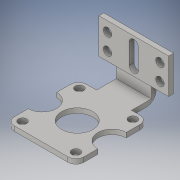
# Autodesk Inventor part: motor mount complete
Saved by Autodesk Inventor 2016 (Build 200138000, 138)
## iProperties
Created: 2017-09-13
Part Number: motor mount complete
Material: Generic
Document SubType Name: Modeling
Designer: student
Density: 1 g/cm^3
Appearance: Default
Author: student
Autodesk Inventor part; units mm, degrees
ref_plane "YZ Plane" through (0, 0, 0) normal (1, 0, 0) x (0, 1, 0)
ref_plane "XZ Plane" through (0, 0, 0) normal (0, 1, 0) x (-1, 0, 0)
ref_plane "XY Plane" through (0, 0, 0) normal (0, 0, 1) x (1, 0, 0)
sketch "Sketch1" plane through (0, 0, 0) normal (0, 0, 1) x (1, 0, 0)
  line L0 (-11.0744, 5.588) -> (11.0744, 5.588)
  line L1 (11.0744, 5.588) -> (11.0744, -5.588)
  line L2 (11.0744, -5.588) -> (-11.0744, -5.588)
  line L3 (-11.0744, -5.588) -> (-11.0744, 5.588)
  circle A0 centre (-8.3312, 2.4384) radius 1.3462
  circle A1 centre (8.3312, 2.4384) radius 1.3462
  circle A2 centre (8.3312, -2.794) radius 1.3462
  circle A3 centre (-8.3312, -2.794) radius 1.3462
  line L4 (0, -3.2143) -> (0, 3.2143) construction
  line L5 (1.4766, -3.2143) -> (1.4766, 3.2143)
  line L6 (-1.4766, 3.2143) -> (-1.4766, -3.2143)
  arc A4 (-1.4766, -3.2143) -> (1.4766, -3.2143) centre (0, -3.2143) ccw
  arc A5 (1.4766, 3.2143) -> (-1.4766, 3.2143) centre (0, 3.2143) ccw
  point P0 (0, 0)
  dimension "d0" = 22.1488
  dimension "d1" = 11.176
  dimension "d2" = 2.6924
  dimension "d3" = 2.6924
  dimension "d4" = 2.6924
  dimension "d5" = 2.6924
  dimension "d6" = 3.1496
  dimension "d7" = 2.794
  dimension "d8" = 5.2324
  dimension "d9" = 2.7432
  dimension "d10" = 2.7432
  dimension "d11" = 3.1496
  dimension "d12" = 2.794
  constraints: 16 end point, 6 centre point, 4 point on circle, 4 tangent, 3 parallel, 2 vertical alignment, 1 horizontal, 1 midpoint, 1 perpendicular, 1 vertical
  measures "d0" distance of L1.end L2.end
  measures "d1" distance of L1.end L0.end
  measures "d2" diameter of A0
  measures "d3" diameter of A1
  measures "d4" diameter of A2
  measures "d5" diameter of A3
  measures "d6" distance from line of L0 A1.centre
  measures "d7" distance from line of L2 A2.centre
  measures "d8" distance of A2.centre A1.centre
  measures "d9" distance from line of L1 A1.centre
  measures "d10" distance from line of L3 A0.centre
  measures "d11" vertical distance of L0.start A0.centre
  measures "d12" distance from line of L2 A3.centre
extrude "Extrusion1" add sketch "Sketch1" along normal blind 1.5494 contours L0 L1 L2 L3 | A4 L6 A5 L5
sketch "Sketch2" plane through (-11.0744, -5.588, 0) normal (0, -1, 0) x (1, 0, 0)
  line L0 (5.5567, 1.5494) -> (16.6565, 1.5494)
  line L1 (16.6565, 1.5494) -> (16.6565, 0)
  line L2 (16.6565, 0) -> (5.5567, 0)
  line L3 (5.5567, 0) -> (5.5567, 1.5494)
  line L4 (22.1488, 0) -> (22.1488, 1.5494) projected
  line L5 (0, 0) -> (0, 1.5494) projected
  line L6 (22.1488, 1.5494) -> (0, 1.5494) projected
  line L7 (0, 0) -> (22.1488, 0) projected
  point P0 (11.0744, 0)
  dimension "d15" = 11.0998
  dimension "d16" = 1.5494
  constraints: 8 end point, 2 parallel, 1 horizontal, 1 perpendicular
  measures "d15" distance of L1.end L2.end
  measures "d16" distance of L1.end L0.end
extrude "Extrusion2" add sketch "Sketch2" along normal blind 3.3782 contours L0 L1 L2 L3
sketch "Sketch3" plane through (-5.5177, -5.588, 1.5494) normal (0, 0, 1) x (1, 0, 0)
  line L0 (0, -3.3559) -> (11.0998, -3.3559)
  line L1 (11.0998, -3.3559) -> (11.0998, -4.8799)
  line L2 (11.0998, -4.8799) -> (0, -4.8799)
  line L3 (0, -4.8799) -> (0, -3.3559)
  point P0 (5.5177, 5.588)
  dimension "d19" = 11.0998
  dimension "d20" = 1.524
  constraints: 8 end point, 2 parallel, 1 horizontal, 1 perpendicular
  measures "d19" distance of L1.end L2.end
  measures "d20" distance of L1.end L0.end
extrude "Extrusion3" add sketch "Sketch3" along normal blind 6.4008
sketch "Sketch4" plane through (-5.5177, -8.9439, 1.5494) normal (0, 1, 0) x (1, 0, 0)
  line L0 (13.7962, -29.1915) -> (-3.1964, -29.1915)
  line L1 (-3.1964, -6.3061) -> (13.7962, -6.3061)
  line L2 (-5.5567, 1.5494) -> (16.5921, 1.5494) projected
  arc A0 (-5.7364, -22.2822) -> (-5.7364, -13.2153) centre (-5.7998, -17.7488) ccw
  arc A1 (16.3362, -13.2152) -> (16.3362, -22.2823) centre (16.3912, -17.7488) ccw
  line L3 (16.3362, -8.8461) -> (16.3362, -13.2152)
  line L4 (16.3362, -22.2823) -> (16.3362, -26.6515)
  line L5 (-5.7364, -26.6515) -> (-5.7364, -22.2822)
  line L6 (-5.7364, -13.2153) -> (-5.7364, -8.8461)
  circle A2 centre (5.2999, -17.7488) radius 4.9657
  arc A3 (13.7962, -29.1915) -> (16.3362, -26.6515) centre (13.7962, -26.6515) ccw
  arc A4 (-5.7364, -26.6515) -> (-3.1964, -29.1915) centre (-3.1964, -26.6515) ccw
  arc A5 (16.3362, -8.8461) -> (13.7962, -6.3061) centre (13.7962, -8.8461) ccw
  arc A6 (-3.1964, -6.3061) -> (-5.7364, -8.8461) centre (-3.1964, -8.8461) ccw
  circle A7 centre (13.7962, -26.6515) radius 1.3208
  circle A8 centre (13.7962, -8.5679) radius 1.3208
  circle A9 centre (-3.1964, -8.5679) radius 1.3208
  circle A10 centre (-3.1964, -26.6515) radius 1.3208
  point P0 (5.5177, 1.5494)
  point P1 (-5.7364, -6.3061)
  point P2 (-5.7364, -29.1915)
  point P3 (16.3362, -6.3061)
  point P4 (5.5177, 1.5494)
  point P5 (16.3362, -17.7488)
  point P6 (5.5177, 1.5494)
  dimension "d25" = 9.0678
  dimension "d26" = 9.0678
  dimension "d27" = 9.9314
  dimension "d28" = 2.54
  dimension "d29" = 2.6416
  dimension "d30" = 2.6416
  dimension "d31" = 2.6416
  dimension "d32" = 2.6416
  dimension "d33" = 2.54
  constraints: 12 end point, 12 point on circle, 11 centre point, 8 tangent, 6 point on line, 5 parallel, 3 equal radius, 3 horizontal alignment, 2 coincident, 2 midpoint, 2 perpendicular, 2 vertical alignment, 1 horizontal
  measures "d25" diameter of A0
  measures "d26" diameter of A1
  measures "d27" diameter of A2
  measures "d28" radius of A3
  measures "d29" diameter of A7
  measures "d30" diameter of A8
  measures "d31" diameter of A9
  measures "d32" diameter of A10
  measures "d33" distance from line of L0 A4.centre
extrude "Extrusion4" add sketch "Sketch4" against normal blind 1.524
sketch "Sketch5" plane through (-11.0744, -8.9662, 0) normal (0, -1, 0) x (1, 0, 0)
  line L0 (16.6565, 1.5494) -> (5.5567, 1.5494) projected
  line L1 (5.5567, 1.5494) -> (5.5567, 0) projected
  line L2 (5.5567, 0) -> (16.6565, 0) projected
  line L3 (16.6565, 0) -> (16.6565, 1.5494) projected
  point P0 (11.0744, 0)
extrude "Extrusion5" add sketch "Sketch5" along normal blind 1.5016
fillet "Fillet1" radius 3.175 1 edges at (0.0322, -10.4678, 0)
sketch "Sketch6" plane through (0, 0, 0) normal (0, 0, -1) x (-1, 0, 0)
  line L0 (0, -3.2139) -> (0, 3.2139) construction
  line L1 (1.4732, -3.2139) -> (1.4732, 3.2139)
  line L2 (-1.4732, 3.2139) -> (-1.4732, -3.2139)
  arc A0 (-1.4732, -3.2139) -> (1.4732, -3.2139) centre (0, -3.2139) ccw
  arc A1 (1.4732, 3.2139) -> (-1.4732, 3.2139) centre (0, 3.2139) ccw
  point P0 (0, 0)
  dimension "d41" = 2.9464
  constraints: 8 end point, 4 point on circle, 4 tangent, 2 centre point, 1 midpoint, 1 parallel, 1 vertical
  measures "d41" diameter of A1
extrude "Extrusion6" cut sketch "Sketch6" against normal blind 9.4615
equation "\"BendRadius\" = Thickness"
equation "\"BendReliefWidth\" = Thickness"
equation "\"BendReliefDepth\" = 0.5 * Thickness"
equation "\"CornerReliefSize\" = 4 * Thickness"
equation "\"MinimumRemnant\" = 2 * Thickness"
equation "\"TransitionRadius\" = BendRadius"
equation "\"JacobiRadiusSize\" = Thickness"
equation "\"GapSize\" = Thickness"
equation "\"Thickness\" = 3.048"
body "Solid1"
